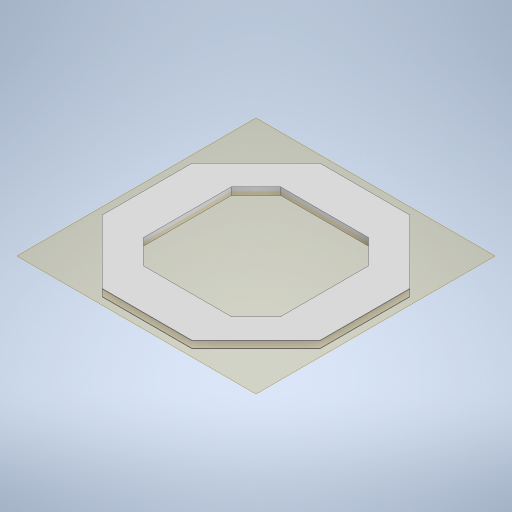
# Autodesk Inventor part: 팔각형 OV-PAM 층 한개
Saved by Autodesk Inventor 2024 (Build 280153000, 153)
## iProperties
Created: 2023-06-16
Part Number: 팔각형 OV-PAM 층 한개
Material: 일반
Document SubType Name: Modeling
Designer: jsw
Density: 1 g/cm^3
Appearance: 기본값
Mass: 0.294629 g
Surface Area: 85.2558 cm^2
Volume: 0.294629 cm^3
Author: jsw
Autodesk Inventor part; units mm, degrees
ref_plane "YZ Plane" through (0, 0, 0) normal (1, 0, 0) x (0, 1, 0)
ref_plane "XZ Plane" through (0, 0, 0) normal (0, 1, 0) x (-1, 0, 0)
ref_plane "XY Plane" through (0, 0, 0) normal (0, 0, 1) x (1, 0, 0)
sketch "스케치1" plane through (0, 0, 0) normal (0, 1, 0) x (-1, 0, 0)
  line L0 (-32.5919, 13.5) -> (-13.5, 32.5919)
  line L1 (-13.5, 32.5919) -> (13.5, 32.5919)
  line L2 (13.5, 32.5919) -> (32.5919, 13.5)
  line L3 (32.5919, 13.5) -> (32.5919, -13.5)
  line L4 (32.5919, -13.5) -> (13.5, -32.5919)
  line L5 (13.5, -32.5919) -> (-13.5, -32.5919)
  line L6 (-13.5, -32.5919) -> (-32.5919, -13.5)
  line L7 (-32.5919, -13.5) -> (-32.5919, 13.5)
  line L8 (-13.8314, 33.3919) -> (13.8314, 33.3919)
  line L9 (13.8314, 33.3919) -> (33.3919, 13.8314)
  line L10 (33.3919, 13.8314) -> (33.3919, -13.8314)
  line L11 (33.3919, -13.8314) -> (13.8314, -33.3919)
  line L12 (13.8314, -33.3919) -> (-13.8314, -33.3919)
  line L13 (-13.8314, -33.3919) -> (-33.3919, -13.8314)
  line L14 (-33.3919, -13.8314) -> (-33.3919, 13.8314)
  line L15 (-33.3919, 13.8314) -> (-13.8314, 33.3919)
  point P0 (0, 0)
  point P1 (0, 0)
  point P2 (0, 0)
  dimension "d0" = 27
  dimension "d2" = 0.8
  constraints: 32 end point, 2 coincident, 2 horizontal, 34 other
  measures "d0" distance of L0.end L1.end
  measures "d2" distance between parallel lines of L10 L3
extrude "돌출2" add sketch "스케치1" along normal blind 2.2688 contours L0 L1 L2 L3 L4 L5 L6 L7 | L8 L9 L10 L11 L12 L13 L14 L15
ref_plane "작업 평면5" through (0, 1.1344, 0) normal (0, 1, 0) x (1, 0, 0)
sketch "스케치9" plane through (0, 1.1344, 0) normal (0, 1, 0) x (1, 0, 0)
  line L0 (-13.8314, 21.8449) -> (13.8314, 21.8449)
  line L1 (13.8314, 33.3919) -> (-13.8314, 33.3919) projected
  line L2 (-13.8314, -21.8449) -> (13.8314, -21.8449)
  line L3 (21.8449, 13.8314) -> (21.8449, -13.8314)
  line L4 (-21.8449, 13.8314) -> (-21.8449, -13.8314)
  line L5 (33.3919, -13.8314) -> (33.3919, 13.8314) projected
  line L6 (-33.3919, 13.8314) -> (-33.3919, -13.8314) projected
  line L7 (-13.8314, -33.3919) -> (13.8314, -33.3919) projected
  line L8 (13.8314, -21.8449) -> (21.8449, -13.8314)
  line L9 (21.8449, 13.8314) -> (13.8314, 21.8449)
  line L10 (-13.8314, 21.8449) -> (-21.8449, 13.8314)
  line L11 (-21.8449, -13.8314) -> (-13.8314, -21.8449)
  line L12 (33.3919, -13.8314) -> (33.3919, 13.8314) projected
  line L13 (13.8314, -33.3919) -> (33.3919, -13.8314) projected
  line L14 (-13.8314, -33.3919) -> (13.8314, -33.3919) projected
  line L15 (-33.3919, -13.8314) -> (-13.8314, -33.3919) projected
  line L16 (-33.3919, 13.8314) -> (-33.3919, -13.8314) projected
  line L17 (-13.8314, 33.3919) -> (-33.3919, 13.8314) projected
  line L18 (13.8314, 33.3919) -> (-13.8314, 33.3919) projected
  line L19 (33.3919, 13.8314) -> (13.8314, 33.3919) projected
  point P0 (33.3919, 13.8314)
  point P1 (-13.8314, 33.3919)
  point P2 (-33.3919, -13.8314)
  dimension "d38" = 11.547
  dimension "d39" = 11.547
  dimension "d40" = 11.547
  dimension "d41" = 11.547
  constraints: 16 end point, 4 horizontal alignment, 4 vertical alignment, 2 horizontal, 2 vertical, 1 perpendicular
  measures "d38" distance between parallel lines of L0 L1
  measures "d39" distance between parallel lines of L5 L3
  measures "d40" distance between parallel lines of L6 L4
  measures "d41" distance between parallel lines of L7 L2
extrude "돌출8" cut sketch "스케치9" along normal mid plane 2
shell "쉘6" thickness 0.8 removed faces 2 at (11.1306, 2.2688, 4.6105) at (11.1306, 0, 4.6105)
